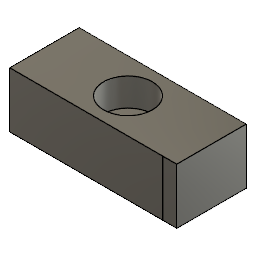
Endstop Y Motor (Autodesk Fusion 360 design; units mm, degrees)
Autodesk Fusion 360 part; units mm, degrees
sketch "Skizze1" plane through (0, 0, 0) normal (0, 1, 0) x (1, 0, 0)
  line L0 (0, 0) -> (20, 0)
  line L1 (20, 0) -> (20, -10)
  line L2 (20, -10) -> (0, -10)
  line L3 (0, 0) -> (0, -10)
  constraint coincident L0.start L3.start
  constraint horizontal L0
  constraint perpendicular L0 L1
  constraint perpendicular L1 L2
  constraint perpendicular L2 L3
extrude "Extrusion1" add sketch "Skizze1" along normal blind 8
sketch "Skizze2" plane through (0, 8, 0) normal (0, 1, 0) x (-1, 0, 0)
  line L0 (-20, 0) -> (0, 0)
  line L1 (0, 0) -> (0, 10)
  line L2 (0, 10) -> (-20, 10)
  line L3 (-20, 10) -> (-20, 0)
  line L4 (0, 0) -> (0, 5)
  circle A0 centre (-10, 5) radius 1.275
  dimension "d3" = 2.55
  constraint coincident L0.end L1.start
  constraint midpoint L1 L4.end
  measures "d3" diameter of A0
extrude "Extrusion2" cut sketch "Skizze2" against normal blind 24 contours A0
sketch "Skizze3" plane through (0, 8, 0) normal (0, 1, 0) x (-1, 0, 0)
  circle A0 centre (-10, 5) radius 1.275
  line L0 (-20, 0) -> (0, 0)
  line L1 (0, 0) -> (0, 10)
  line L2 (0, 10) -> (-20, 10)
  line L3 (-20, 10) -> (-20, 0)
  circle A1 centre (-10, 5) radius 3.5
  dimension "d6" = 7
  constraint concentric A0 A1
  measures "d6" diameter of A1
extrude "Extrusion3" cut sketch "Skizze3" against normal blind 4 contours A1
sketch "Skizze4" plane through (0, 8, 0) normal (0, 1, 0) x (-1, 0, 0)
  circle A0 centre (-10, 5) radius 3.5
  line L0 (-20, 0) -> (0, 0)
  line L1 (0, 0) -> (0, 10)
  line L2 (0, 10) -> (-20, 10)
  line L3 (-20, 10) -> (-20, 0)
  line L4 (0, 0) -> (0, 5)
  line L5 (0, 0) -> (0, 10)
  line L6 (0, 10) -> (2, 10)
  line L7 (2, 10) -> (2, 0)
  line L8 (2, 0) -> (0, 0)
  line L9 (-20, 0) -> (-22, 0)
  line L10 (-22, 0) -> (-22, 10)
  line L11 (-22, 10) -> (-20, 10)
  constraint coincident L0.end L1.start
  constraint midpoint L1 L4.end
  constraint coincident L1.end L2.start
  constraint perpendicular L5 L6
  constraint perpendicular L6 L7
  constraint perpendicular L7 L8
  constraint coincident L0.start L3.end
  constraint perpendicular L3 L9
  constraint perpendicular L9 L10
  constraint coincident L2.end L3.start
extrude "Extrusion4" add sketch "Skizze4" against normal blind 8 contours L3 L9 L10 L11 | L1 L4 L5 L6 L7 L8
sketch "Skizze5" plane through (0, 8, 0) normal (0, 1, 0) x (-1, 0, 0)
  circle A0 centre (-10, 5) radius 3.5
  line L0 (-22, 0) -> (2, 0)
  line L1 (2, 0) -> (2, 10)
  line L2 (2, 10) -> (-20, 10)
  line L3 (-20, 10) -> (-22, 10)
  line L4 (-22, 10) -> (-22, 0)
  line L5 (2, 0) -> (2, 5)
  line L6 (2, 5) -> (0, 5)
  circle A1 centre (0, 5) radius 1.275
  line L7 (-22, 0) -> (-22, 5)
  line L8 (-22, 5) -> (-20, 5)
  circle A2 centre (-20, 5) radius 1.275
  dimension "d11" = 2.55
  dimension "d12" = 2.55
  constraint coincident L0.end L1.start
  constraint midpoint L1 L5.end
  constraint perpendicular L1 L6
  constraint coincident L6.end A1.centre
  constraint coincident L0.start L4.end
  constraint midpoint L4 L7.end
  constraint perpendicular L4 L8
  constraint coincident L8.end A2.centre
  measures "d11" diameter of A1
  measures "d12" diameter of A2
extrude "Extrusion5" cut sketch "Skizze5" against normal blind 4 contours A1 | A2
delete_face "Fläche löschen1" 1 faces at (18.7313, 6.6667, 5.1269)
delete_face "Fläche löschen2" 1 faces at (-1.2687, 6.6667, 4.8731)
